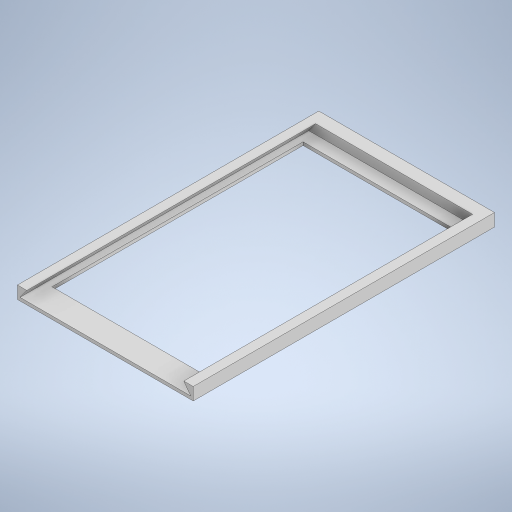
# Autodesk Inventor part: cover
Saved by Autodesk Inventor 2023 (Build 270158000, 158)
## iProperties
Created: 2023-03-10
Part Number: cover
Material: Типовые
Document SubType Name: Modeling
Designer: Josh
Density: 1 g/cm^3
Appearance: По умолчанию
Author: Josh
Autodesk Inventor part; units mm, degrees
ref_plane "YZ Plane" through (0, 0, 0) normal (1, 0, 0) x (0, 1, 0)
ref_plane "XZ Plane" through (0, 0, 0) normal (0, 1, 0) x (-1, 0, 0)
ref_plane "XY Plane" through (0, 0, 0) normal (0, 0, 1) x (1, 0, 0)
sketch "Эскиз1" plane through (0, 0, 0) normal (0, 1, 0) x (-1, 0, 0)
  line L0 (-25, -40) -> (25, -40)
  line L1 (25, -40) -> (25, 40)
  line L2 (25, 40) -> (-25, 40)
  line L3 (-25, 40) -> (-25, -40)
  line L4 (-25, -40) -> (25, 40) construction
  line L5 (25, -40) -> (-25, 40) construction
  line L6 (28, 43) -> (28, -43)
  line L7 (28, -43) -> (-28, -43)
  line L8 (-28, -43) -> (-28, 43)
  line L9 (-28, 43) -> (28, 43)
  line L10 (28, 43) -> (25, 43)
  line L11 (25, 43) -> (25, -43)
  line L12 (25, -43) -> (28, -43)
  line L13 (28, -43) -> (28, 43)
  line L14 (-28, 43) -> (-25, 43)
  line L15 (-25, 43) -> (-25, -43)
  line L16 (-25, -43) -> (-28, -43)
  line L17 (-28, -43) -> (-28, 43)
  point P0 (0, 0)
  point P1 (-25, 43)
  dimension "d0" = 50
  dimension "d1" = 80
  dimension "d2" = 3
  constraints: 36 end point, 8 parallel, 4 perpendicular, 3 horizontal, 2 midpoint, 2 point on line, 3 other
  measures "d0" distance of L2.end L1.end
  measures "d1" distance of L1.end L0.end
  measures "d2" distance between parallel lines of L1 L6
extrude "Выдавливание1" add sketch "Эскиз1" along normal blind 1 contours L15 L7 L8 L9 L3 | L0 L11 L7 L15 | L1 L11 L9 L6 L7 | L15 L9 L11 L2
extrude "Выдавливание2" add sketch "Эскиз1" along normal blind 4 contours L15 L7 L8 L9 L3 | L0 L11 L7 L15 | L1 L11 L9 L6 L7
sketch "Эскиз2" plane through (-28, 0, 43) normal (0, 0, 1) x (1, 0, 0)
  line L0 (0, 0) -> (0, 4) projected
  line L1 (0, 1) -> (56, 1)
  line L2 (56, 0) -> (56, 4) projected
  line L3 (3, 0) -> (3, 4) projected
  line L4 (3, 4) -> (0.8, 1)
  line L5 (28, 0) -> (28, 4)
  line L6 (53, 4) -> (55.2, 1)
  line L7 (53, 0) -> (53, 4) projected
  line L8 (53, 4) -> (53, 1)
  point P0 (55.2, 1)
  point P1 (3, 1)
  dimension "d7" = 0.8
  constraints: 10 end point, 4 point on line, 2 symmetric about line, 1 collinear, 1 horizontal, 1 vertical
  measures "d7" distance of L4.end L1.start
extrude "Выдавливание3" cut sketch "Эскиз2" against normal up to surface (83 mm away)
sketch "Эскиз3" plane through (-25, 0, -40) normal (0, 0, 1) x (1, 0, 0)
  line L0 (0, 0) -> (50, 0) projected
  line L1 (50, 0) -> (50, 1) projected
  line L2 (52.2, 1) -> (50, 1) projected
  line L3 (50, 4) -> (52.2, 1) projected
  line L4 (0, 4) -> (50, 4) projected
  line L5 (-2.2, 1) -> (0, 4) projected
  line L6 (0, 1) -> (-2.2, 1) projected
  line L7 (0, 0) -> (0, 1) projected
  line L8 (-2.2, 1) -> (52.2, 1) projected
  point P0 (25, 0)
extrude "Выдавливание4" cut sketch "Эскиз3" against normal blind 1 contours L6 L5 L4 L3 L2 L8
sketch "Эскиз4" plane through (28, 0, -43) normal (0, 0, -1) x (-1, 0, 0)
  line L0 (0, 0) -> (56, 0) projected
  line L1 (56, 0) -> (56, 4) projected
  line L2 (0, 4) -> (56, 4) projected
  line L3 (0, 0) -> (0, 4) projected
  point P0 (28, 0)
extrude "Выдавливание5" add sketch "Эскиз4" along normal blind 5
sketch "Эскиз5" plane through (-28, 0, 43) normal (0, 0, 1) x (1, 0, 0)
  line L0 (0.8, 1) -> (55.2, 1) projected
  line L1 (0.8, 1) -> (3, 4) projected
  line L2 (0, 4) -> (3, 4) projected
  line L3 (0, 0) -> (0, 4) projected
  line L4 (0, 0) -> (56, 0) projected
  line L5 (56, 0) -> (56, 4) projected
  line L6 (53, 4) -> (56, 4) projected
  line L7 (53, 4) -> (55.2, 1) projected
  point P0 (28, 0)
extrude "Выдавливание6" add sketch "Эскиз5" along normal blind 5
sketch "Эскиз6" plane through (-25, 0, -41) normal (0, 0, 1) x (1, 0, 0)
  line L0 (0, 4) -> (50, 4) projected
  line L1 (-2.2, 1) -> (0, 4) projected
  line L2 (52.2, 1) -> (-2.2, 1) projected
  line L3 (50, 4) -> (52.2, 1) projected
  point P0 (25, 0)
extrude "Выдавливание7" cut sketch "Эскиз6" against normal blind 3
